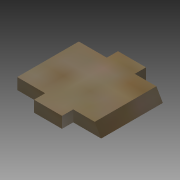
# Autodesk Inventor part: innanverdurstubbur
Saved by Autodesk Inventor 2015 (Build 190159000, 159)
## iProperties
Created: 2015-10-07
Part Number: innanverdurstubbur
Material: Generic
Document SubType Name: Modeling
Designer: Haukur
Density: 1 g/cm^3
Appearance: Plywood - Weathered
Author: Haukur
Autodesk Inventor part; units mm, degrees
ref_plane "YZ Plane" through (0, 0, 0) normal (1, 0, 0) x (0, 1, 0)
ref_plane "XZ Plane" through (0, 0, 0) normal (0, 1, 0) x (-1, 0, 0)
ref_plane "XY Plane" through (0, 0, 0) normal (0, 0, 1) x (1, 0, 0)
sketch "Sketch1" plane through (0, 0, 0) normal (0, 0, 1) x (1, 0, 0)
  line L0 (0, 4) -> (0, 26)
  line L1 (0, 26) -> (10, 26)
  line L2 (10, 26) -> (10, 30)
  line L3 (10, 30) -> (20, 30)
  line L4 (20, 30) -> (20, 26)
  line L5 (20, 26) -> (30, 26)
  line L6 (30, 26) -> (30, 4)
  line L7 (30, 4) -> (20, 4)
  line L8 (20, 4) -> (20, 0)
  line L9 (20, 0) -> (10, 0)
  line L10 (10, 0) -> (10, 4)
  line L11 (10, 4) -> (0, 4)
  point P0 (0, 0)
  dimension "d0" = 22
  dimension "d1" = 10
  dimension "d2" = 4
  dimension "d3" = 10
  dimension "d4" = 10
  constraints: 24 end point, 8 perpendicular, 4 point on line, 1 horizontal, 1 vertical
  measures "d0" distance of L0.start L0.end
  measures "d1" distance of L0.end L1.end
  measures "d2" distance of L1.end L2.end
  measures "d3" distance of L2.end L3.end
  measures "d4" distance of L4.end L5.end
extrude "Extrusion1" add sketch "Sketch1" along normal blind 4
sketch "Sketch2" plane through (20, 26, 0) normal (0, 1, 0) x (1, 0, 0)
  line L0 (10, 0) -> (7.6906, -4)
  line L1 (0, -4) -> (10, -4) projected
  line L2 (10, 0) -> (14.6188, 0) construction
  line L3 (7.6906, -4) -> (10, -4)
  line L4 (10, -4) -> (10, 0)
  point P0 (-20, 0)
  dimension "d7" = 120
  constraints: 8 end point, 1 collinear, 1 equal length, 1 horizontal, 1 perpendicular, 1 point on line
  measures "d7" angle of L0 L2
extrude "Extrusion2" cut sketch "Sketch2" against normal through all
body "Solid1"
